Autodesk Inventor part; units mm, degrees
(part 2 of 2)
  line L108 (12.621, 74.7833) -> (12.5043, 74.7833)
  spline S45 degree 3 poles (12.5043, 74.7833) (12.5014, 74.7709) (12.4959, 74.7471) (12.4838, 74.7136) (12.469, 74.6838) (12.4514, 74.6572) (12.4304, 74.634) (12.4064, 74.6134) (12.3796, 74.5947) (12.3497, 74.5792) (12.3182, 74.5659) (12.2852, 74.5571) (12.2517, 74.5509) (12.229, 74.5503) (12.2176, 74.55) knots 0 0 0 0 0.094687 0.181994 0.264377 0.34218 0.418618 0.496509 0.577369 0.661511 0.746733 0.831258 0.915206 1 1 1 1
  spline S46 degree 3 poles (12.2176, 74.55) (12.2065, 74.5503) (12.1846, 74.5509) (12.1523, 74.5555) (12.1212, 74.5626) (12.0915, 74.5733) (12.0627, 74.5862) (12.0355, 74.6028) (12.0091, 74.6219) (11.9845, 74.6438) (11.9619, 74.668) (11.9419, 74.6938) (11.9253, 74.7213) (11.9113, 74.7501) (11.9006, 74.7804) (11.893, 74.8122) (11.8886, 74.8454) (11.888, 74.8681) (11.8876, 74.8797) knots 0 0 0 0 0.064207 0.126425 0.18768 0.248216 0.308305 0.369661 0.431699 0.495947 0.559758 0.622295 0.683911 0.745092 0.80674 0.869087 0.93329 1 1 1 1
  spline S47 degree 3 poles (11.8876, 74.8797) (11.8879, 74.8901) (11.8884, 74.9105) (11.8923, 74.9404) (11.8991, 74.9686) (11.9085, 74.9954) (11.9205, 75.0208) (11.9352, 75.0447) (11.9528, 75.0669) (11.9728, 75.0873) (11.9949, 75.1062) (12.0192, 75.1223) (12.0453, 75.1359) (12.0728, 75.1475) (12.1025, 75.1559) (12.1338, 75.1622) (12.1669, 75.1659) (12.1895, 75.1664) (12.2012, 75.1666) knots 0 0 0 0 0.065351 0.127916 0.18836 0.247216 0.30563 0.36377 0.422661 0.482687 0.5433 0.604118 0.664965 0.727413 0.791468 0.858055 0.927037 1 1 1 1
  spline S48 degree 3 poles (12.2012, 75.1666) (12.2113, 75.1664) (12.2321, 75.166) (12.264, 75.1627) (12.2975, 75.1574) (12.3325, 75.1501) (12.3692, 75.1406) (12.4073, 75.1292) (12.4471, 75.1156) (12.4739, 75.1053) (12.4876, 75.1) knots 0 0 0 0 0.102203 0.211023 0.3251 0.446502 0.573788 0.708901 0.850358 1 1 1 1
  line L109 (9.041, 74.45) -> (8.4243, 75.75)
  line L110 (8.4243, 75.75) -> (8.4076, 75.75)
  line L111 (8.4076, 75.75) -> (7.8076, 74.45)
  line L112 (7.8076, 74.45) -> (7.9345, 74.45)
  line L113 (7.9345, 74.45) -> (8.1267, 74.8666)
  line L114 (8.1267, 74.8666) -> (8.716, 74.8666)
  line L115 (8.716, 74.8666) -> (8.9136, 74.45)
  line L116 (8.9136, 74.45) -> (9.041, 74.45)
  spline S49 degree 3 poles (7.531, 75.1075) (7.5304, 75.1309) (7.5293, 75.1769) (7.5196, 75.2444) (7.5041, 75.3091) (7.482, 75.3709) (7.454, 75.43) (7.4195, 75.486) (7.3788, 75.5393) (7.3322, 75.5891) (7.2811, 75.6346) (7.2263, 75.6746) (7.1681, 75.708) (7.107, 75.7358) (7.0426, 75.7572) (6.9749, 75.7722) (6.9042, 75.7815) (6.856, 75.7827) (6.8315, 75.7833) knots 0 0 0 0 0.064558 0.127014 0.187955 0.248014 0.307748 0.368235 0.42947 0.492743 0.556258 0.618217 0.679655 0.741246 0.803415 0.866815 0.932328 1 1 1 1
  spline S50 degree 3 poles (6.8315, 75.7833) (6.8166, 75.7831) (6.787, 75.7828) (6.7433, 75.7793) (6.7007, 75.7736) (6.6592, 75.7657) (6.6187, 75.756) (6.5794, 75.7433) (6.5411, 75.7288) (6.5041, 75.7121) (6.4684, 75.6934) (6.4342, 75.6728) (6.4017, 75.6504) (6.3707, 75.6264) (6.3417, 75.6002) (6.3139, 75.5727) (6.2882, 75.5429) (6.2723, 75.5219) (6.2643, 75.5114) knots 0 0 0 0 0.068548 0.135683 0.201215 0.265682 0.329267 0.392395 0.45507 0.517127 0.57879 0.63974 0.700192 0.759806 0.819628 0.879355 0.939512 1 1 1 1
  line L117 (6.2643, 75.5114) -> (6.3664, 75.4333)
  spline S51 degree 3 poles (6.3664, 75.4333) (6.3737, 75.442) (6.3881, 75.4592) (6.4114, 75.4834) (6.4357, 75.5061) (6.4609, 75.5274) (6.4876, 75.5465) (6.515, 75.5644) (6.5437, 75.5805) (6.5833, 75.6) (6.6352, 75.6203) (6.7005, 75.6374) (6.7686, 75.6482) (6.8151, 75.6494) (6.8388, 75.65) knots 0 0 0 0 0.063163 0.125475 0.187121 0.248294 0.309295 0.36985 0.430973 0.492456 0.616148 0.740844 0.868183 1 1 1 1
  spline S52 degree 3 poles (6.8388, 75.65) (6.8518, 75.6498) (6.8778, 75.6495) (6.9163, 75.6456) (6.954, 75.6401) (6.9911, 75.6318) (7.0273, 75.6214) (7.063, 75.609) (7.0976, 75.5937) (7.1317, 75.5767) (7.1643, 75.5575) (7.1951, 75.5366) (7.2241, 75.5142) (7.2512, 75.4902) (7.2766, 75.4647) (7.2999, 75.4374) (7.3211, 75.4085) (7.3407, 75.3783) (7.3582, 75.3469) (7.3729, 75.3142) (7.3859, 75.2807) (7.3962, 75.2461) (7.4043, 75.2106) (7.41, 75.1742) (7.4139, 75.1368) (7.4142, 75.1114) (7.4143, 75.0987) knots 0 0 0 0 0.043955 0.087502 0.130463 0.172752 0.215403 0.25765 0.300153 0.343121 0.385925 0.427686 0.468818 0.509492 0.549883 0.58998 0.630405 0.670869 0.711384 0.751627 0.791776 0.832459 0.873319 0.914543 0.956924 1 1 1 1
  spline S53 degree 3 poles (7.4143, 75.0987) (7.4138, 75.0795) (7.4129, 75.0417) (7.4047, 74.9865) (7.3923, 74.9335) (7.3736, 74.8833) (7.3506, 74.835) (7.3216, 74.7896) (7.2879, 74.7464) (7.2492, 74.7063) (7.2067, 74.6697) (7.1611, 74.6375) (7.1125, 74.6106) (7.0615, 74.5883) (7.0076, 74.5711) (6.951, 74.559) (6.8918, 74.5511) (6.8513, 74.5504) (6.8307, 74.55) knots 0 0 0 0 0.064323 0.12629 0.186726 0.246146 0.305576 0.365429 0.426326 0.48884 0.551725 0.613919 0.675484 0.737334 0.800229 0.864502 0.931041 1 1 1 1
  spline S54 degree 3 poles (6.8307, 74.55) (6.808, 74.5506) (6.7634, 74.5518) (6.6978, 74.5623) (6.6351, 74.5793) (6.5752, 74.603) (6.5183, 74.6338) (6.4642, 74.6712) (6.4129, 74.7156) (6.3821, 74.7494) (6.3664, 74.7666) knots 0 0 0 0 0.128515 0.252949 0.374755 0.49594 0.617181 0.740909 0.867811 1 1 1 1
  line L118 (6.3664, 74.7666) -> (6.2643, 74.6893)
  spline S55 degree 3 poles (6.2643, 74.6893) (6.2725, 74.6787) (6.2889, 74.6576) (6.3155, 74.6277) (6.3434, 74.5997) (6.373, 74.5736) (6.4039, 74.5491) (6.4366, 74.5267) (6.4707, 74.5061) (6.5061, 74.4873) (6.5428, 74.4707) (6.5807, 74.4564) (6.6196, 74.4441) (6.6596, 74.4339) (6.7007, 74.426) (6.7428, 74.4208) (6.786, 74.4171) (6.8152, 74.4168) (6.8299, 74.4166) knots 0 0 0 0 0.061674 0.123053 0.183475 0.243727 0.304279 0.364863 0.425946 0.487391 0.54922 0.611144 0.673529 0.736961 0.800785 0.866013 0.932101 1 1 1 1
  spline S56 degree 3 poles (6.8299, 74.4166) (6.8439, 74.4167) (6.8716, 74.4169) (6.9124, 74.4201) (6.9521, 74.4243) (6.9907, 74.4307) (7.0282, 74.4383) (7.0645, 74.4484) (7.0997, 74.4597) (7.1339, 74.4731) (7.167, 74.4881) (7.1989, 74.5051) (7.2296, 74.524) (7.2593, 74.5442) (7.2878, 74.5665) (7.3152, 74.5905) (7.3416, 74.6162) (7.3579, 74.6347) (7.3661, 74.644) knots 0 0 0 0 0.069663 0.13775 0.203917 0.26878 0.332414 0.394754 0.45618 0.516996 0.577396 0.637198 0.696999 0.756756 0.816554 0.876948 0.938132 1 1 1 1
  spline S57 degree 3 poles (7.3661, 74.644) (7.3793, 74.6602) (7.4055, 74.6923) (7.4389, 74.7444) (7.4676, 74.7988) (7.4908, 74.8558) (7.5089, 74.9152) (7.5214, 74.9772) (7.5296, 75.0415) (7.5305, 75.0853) (7.531, 75.1075) knots 0 0 0 0 0.124329 0.247156 0.36878 0.490734 0.613614 0.738958 0.867311 1 1 1 1
  line L119 (4.4583, 75.7) -> (4.6711, 75.7)
  line L120 (4.8587, 74.6) -> (4.4583, 75.7)
  line L121 (4.3587, 74.6) -> (4.8587, 74.6)
  line L122 (3.9583, 75.7) -> (4.3587, 74.6)
  line L123 (3.7455, 75.7) -> (3.9583, 75.7)
  line L124 (4.1458, 74.6) -> (3.7455, 75.7)
  line L125 (3.9458, 74.6) -> (4.1458, 74.6)
  line L126 (4.0186, 74.4) -> (3.9458, 74.6)
  line L127 (5.1443, 74.4) -> (4.0186, 74.4)
  line L128 (4.6711, 75.7) -> (5.1443, 74.4)
  line L129 (9.8343, 74.45) -> (9.851, 74.45)
  line L130 (9.851, 74.45) -> (10.401, 75.75)
  line L131 (10.401, 75.75) -> (10.276, 75.75)
  line L132 (10.276, 75.75) -> (9.8426, 74.7255)
  line L133 (9.8426, 74.7255) -> (9.4093, 75.75)
  line L134 (9.4093, 75.75) -> (9.2843, 75.75)
  line L135 (9.2843, 75.75) -> (9.8343, 74.45)
  spline S58 degree 3 poles (10.6443, 75.0995) (10.6446, 75.0796) (10.645, 75.0408) (10.6475, 74.9842) (10.6523, 74.9307) (10.6583, 74.8803) (10.6666, 74.8331) (10.6769, 74.789) (10.6883, 74.7478) (10.7023, 74.7098) (10.7177, 74.6745) (10.7344, 74.6416) (10.7524, 74.6107) (10.7719, 74.5821) (10.7927, 74.5556) (10.8153, 74.5316) (10.8389, 74.5096) (10.864, 74.4901) (10.8901, 74.473) (10.9168, 74.4577) (10.9446, 74.4453) (10.9728, 74.4347) (11.0018, 74.4266) (11.0316, 74.421) (11.0621, 74.4171) (11.0827, 74.4168) (11.093, 74.4166) knots 0 0 0 0 0.065063 0.126773 0.185516 0.240765 0.29298 0.34225 0.388919 0.432776 0.474628 0.514775 0.553606 0.591426 0.628028 0.663804 0.698984 0.733591 0.767628 0.801208 0.834264 0.866981 0.89972 0.932702 0.966176 1 1 1 1
  spline S59 degree 3 poles (11.093, 74.4166) (11.1033, 74.4168) (11.1235, 74.4172) (11.1534, 74.4207) (11.1825, 74.4264) (11.2109, 74.4343) (11.2386, 74.4441) (11.2654, 74.4568) (11.2915, 74.4714) (11.3168, 74.488) (11.341, 74.5071) (11.3641, 74.5281) (11.3855, 74.5518) (11.4054, 74.5776) (11.4243, 74.6053) (11.4417, 74.6354) (11.4578, 74.6676) (11.4726, 74.7023) (11.4856, 74.7399) (11.4972, 74.7808) (11.5063, 74.8254) (11.5141, 74.8734) (11.5203, 74.9249) (11.5246, 74.98) (11.5273, 75.0386) (11.5275, 75.0788) (11.5276, 75.0995) knots 0 0 0 0 0.033787 0.066622 0.099285 0.131361 0.163585 0.196104 0.228902 0.262158 0.295991 0.330218 0.36506 0.400951 0.43762 0.475708 0.515381 0.556414 0.599765 0.646424 0.696431 0.749782 0.806573 0.867436 0.931887 1 1 1 1
  spline S60 degree 3 poles (11.5276, 75.0995) (11.5275, 75.1203) (11.5273, 75.1608) (11.5247, 75.2197) (11.5203, 75.2751) (11.5143, 75.3268) (11.507, 75.3748) (11.4973, 75.4191) (11.4862, 75.4598) (11.4733, 75.4971) (11.4589, 75.5315) (11.4431, 75.5636) (11.4254, 75.5934) (11.4069, 75.6213) (11.3867, 75.6469) (11.3654, 75.6705) (11.3422, 75.6917) (11.3179, 75.7109) (11.2923, 75.7278) (11.266, 75.7427) (11.239, 75.7554) (11.2111, 75.7654) (11.1826, 75.7736) (11.1534, 75.7793) (11.1235, 75.7828) (11.1033, 75.7831) (11.093, 75.7833) knots 0 0 0 0 0.068595 0.133246 0.194313 0.251279 0.304513 0.354235 0.400481 0.443411 0.484015 0.523252 0.561042 0.5979 0.633518 0.668314 0.702496 0.736685 0.770293 0.803437 0.835913 0.86846 0.900847 0.933467 0.966258 1 1 1 1
  spline S61 degree 3 poles (11.093, 75.7833) (11.0827, 75.7831) (11.0621, 75.7828) (11.0317, 75.7793) (11.002, 75.7736) (10.9731, 75.7654) (10.9449, 75.7553) (10.9174, 75.7427) (10.8906, 75.7279) (10.8648, 75.7106) (10.8399, 75.6913) (10.8163, 75.6695) (10.7941, 75.6453) (10.7731, 75.6192) (10.7538, 75.5905) (10.7353, 75.5597) (10.7189, 75.5264) (10.703, 75.491) (10.6893, 75.4527) (10.6769, 75.4115) (10.6669, 75.3671) (10.6586, 75.3197) (10.6522, 75.269) (10.6475, 75.2152) (10.645, 75.1583) (10.6446, 75.1194) (10.6443, 75.0995) knots 0 0 0 0 0.033788 0.067194 0.099862 0.132567 0.165151 0.197913 0.231319 0.265083 0.299255 0.334399 0.369943 0.406284 0.444064 0.482998 0.523354 0.565537 0.609613 0.656391 0.705885 0.758325 0.813832 0.872795 0.934722 1 1 1 1
  line L136 (16.7943, 75.1) -> (16.661, 75.75)
  line L137 (16.661, 75.75) -> (16.1276, 75.75)
  line L138 (16.1276, 75.75) -> (16.1276, 75.6166)
  line L139 (16.1276, 75.6166) -> (16.5698, 75.6166)
  line L140 (16.5698, 75.6166) -> (16.6399, 75.2747)
  spline S62 degree 3 poles (16.6399, 75.2747) (16.6261, 75.2785) (16.5995, 75.2859) (16.5601, 75.2941) (16.5227, 75.299) (16.4985, 75.2997) (16.4868, 75.3) knots 0 0 0 0 0.275068 0.532901 0.773973 1 1 1 1
  spline S63 degree 3 poles (16.4868, 75.3) (16.4722, 75.2997) (16.4437, 75.299) (16.4019, 75.2931) (16.3621, 75.2838) (16.3242, 75.2707) (16.2882, 75.2541) (16.2545, 75.2332) (16.2225, 75.2089) (16.1928, 75.1809) (16.1658, 75.1501) (16.1422, 75.117) (16.122, 75.0819) (16.1059, 75.0444) (16.0929, 75.0051) (16.0843, 74.9634) (16.0786, 74.9198) (16.078, 74.8899) (16.0776, 74.8747) knots 0 0 0 0 0.065808 0.129394 0.190894 0.251281 0.310815 0.370371 0.430768 0.492881 0.555104 0.616067 0.677256 0.73826 0.800762 0.864778 0.931045 1 1 1 1
  spline S64 degree 3 poles (16.0776, 74.8747) (16.0779, 74.8641) (16.0784, 74.8431) (16.0809, 74.8118) (16.0857, 74.7812) (16.0921, 74.7513) (16.1005, 74.7221) (16.1106, 74.6935) (16.123, 74.6657) (16.1367, 74.6385) (16.152, 74.6124) (16.169, 74.588) (16.1869, 74.565) (16.2063, 74.5435) (16.2271, 74.5237) (16.2493, 74.5055) (16.2726, 74.4886) (16.2974, 74.4737) (16.323, 74.46) (16.35, 74.4487) (16.3777, 74.4386) (16.4064, 74.4306) (16.4361, 74.4243) (16.467, 74.4201) (16.4987, 74.4169) (16.5202, 74.4167) (16.531, 74.4166) knots 0 0 0 0 0.044014 0.087434 0.130118 0.172554 0.214555 0.256298 0.298438 0.340849 0.382715 0.423924 0.464246 0.504074 0.543862 0.583567 0.623094 0.663229 0.703551 0.743938 0.784541 0.82575 0.867757 0.910745 0.954914 1 1 1 1
  spline S65 degree 3 poles (16.531, 74.4166) (16.544, 74.4169) (16.5695, 74.4174) (16.6068, 74.4227) (16.6427, 74.4303) (16.6769, 74.4416) (16.7098, 74.4559) (16.7408, 74.4739) (16.7707, 74.4943) (16.7984, 74.5184) (16.8241, 74.5448) (16.847, 74.5734) (16.8675, 74.6037) (16.8852, 74.636) (16.9002, 74.6701) (16.912, 74.7062) (16.9216, 74.744) (16.9256, 74.7701) (16.9276, 74.7833) knots 0 0 0 0 0.065421 0.128708 0.190236 0.250724 0.310637 0.370766 0.431615 0.493523 0.555883 0.617342 0.678668 0.740711 0.802985 0.866803 0.932347 1 1 1 1
  line L141 (16.9276, 74.7833) -> (16.811, 74.7833)
  spline S66 degree 3 poles (16.811, 74.7833) (16.8081, 74.7709) (16.8026, 74.7471) (16.7905, 74.7136) (16.7757, 74.6838) (16.7581, 74.6572) (16.7371, 74.634) (16.7131, 74.6134) (16.6862, 74.5947) (16.6564, 74.5792) (16.6249, 74.5659) (16.5919, 74.5571) (16.5583, 74.5509) (16.5357, 74.5503) (16.5243, 74.55) knots 0 0 0 0 0.094687 0.181994 0.264377 0.34218 0.418618 0.496509 0.577369 0.661511 0.746733 0.831258 0.915206 1 1 1 1
  spline S67 degree 3 poles (16.5243, 74.55) (16.5131, 74.5503) (16.4912, 74.5509) (16.459, 74.5555) (16.4278, 74.5626) (16.3981, 74.5733) (16.3693, 74.5862) (16.3421, 74.6028) (16.3158, 74.6219) (16.2911, 74.6438) (16.2685, 74.668) (16.2486, 74.6938) (16.2319, 74.7213) (16.2179, 74.7501) (16.2073, 74.7804) (16.1997, 74.8122) (16.1952, 74.8454) (16.1946, 74.8681) (16.1943, 74.8797) knots 0 0 0 0 0.064207 0.126425 0.18768 0.248216 0.308305 0.369661 0.431699 0.495947 0.559758 0.622295 0.683911 0.745092 0.80674 0.869087 0.93329 1 1 1 1
  spline S68 degree 3 poles (16.1943, 74.8797) (16.1946, 74.8901) (16.195, 74.9105) (16.1989, 74.9404) (16.2057, 74.9686) (16.2152, 74.9954) (16.2272, 75.0208) (16.2418, 75.0447) (16.2594, 75.0669) (16.2795, 75.0873) (16.3015, 75.1062) (16.3258, 75.1223) (16.3519, 75.1359) (16.3795, 75.1475) (16.4092, 75.1559) (16.4404, 75.1622) (16.4736, 75.1659) (16.4962, 75.1664) (16.5079, 75.1666) knots 0 0 0 0 0.065351 0.127916 0.18836 0.247216 0.30563 0.36377 0.422661 0.482687 0.5433 0.604118 0.664965 0.727413 0.791468 0.858055 0.927037 1 1 1 1
  spline S69 degree 3 poles (16.5079, 75.1666) (16.5179, 75.1664) (16.5387, 75.166) (16.5706, 75.1627) (16.6042, 75.1574) (16.6392, 75.1501) (16.6758, 75.1406) (16.714, 75.1292) (16.7538, 75.1156) (16.7805, 75.1053) (16.7943, 75.1) knots 0 0 0 0 0.102203 0.211023 0.3251 0.446502 0.573788 0.708901 0.850358 1 1 1 1
  line L142 (0, 0) -> (0, 80)
  point P0 (43, 40)
  point P1 (5.1443, 7.8)
  point P2 (5.1443, 72.2)
  constraints: 284 end point, 140 symmetric about line, 60 point on circle, 36 horizontal, 34 centre point, 1 midpoint, 161 other
extrude "Выдавливание32" cut sketch "Эскиз43" against normal blind 5 contours A16 | A33
equation "\"d3\" = d2"
equation "\"d5\" = d4"
equation "\"d6\" = d2"
equation "\"d7\" = d2"
equation "\"d9\" = d8"
equation "\"d10\" = d8"
equation "\"d11\" = d8"
equation "\"d17\" = d14"
equation "\"d18\" = d16"
equation "\"d19\" = d14"
equation "\"d21\" = d16"
equation "\"d22\" = d16"
equation "\"d23\" = d14"
